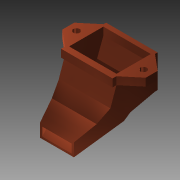
# Autodesk Inventor part: dysza_abs2
Saved by Autodesk Inventor 2013 (Build 170138000, 138)
## iProperties
Created: 2013-08-26
Part Number: dysza_abs2
Material: Generic
Document SubType Name: Modeling
Designer: dzban
Density: 1 g/cm^3
Author: dzban
Autodesk Inventor part; units mm, degrees
ref_plane "YZ Plane" through (0, 0, 0) normal (1, 0, 0) x (0, 1, 0)
ref_plane "XZ Plane" through (0, 0, 0) normal (0, 1, 0) x (-1, 0, 0)
ref_plane "XY Plane" through (0, 0, 0) normal (0, 0, 1) x (1, 0, 0)
sketch "Sketch1" plane through (0, 0, 0) normal (1, 0, 0) x (0, 1, 0)
  line L0 (0, 0) -> (15, 0)
  line L1 (15, 0) -> (12.3428, -7.0424)
  line L2 (12.3428, -7.0424) -> (2.9628, -13.5)
  line L3 (2.9628, -13.5) -> (-16.504, -16)
  line L4 (-16.504, -16) -> (-16.504, -11)
  line L5 (-16.504, -11) -> (-7.6685, -9.267)
  line L6 (-7.6685, -9.267) -> (-2.3251, -6.639)
  line L7 (-2.3251, -6.639) -> (0, 0)
  dimension "d0" = 15
  dimension "d24" = 16
  dimension "d27" = 5
  constraints: 16 end point, 1 horizontal, 1 vertical
  measures "d0" distance of L0.start L0.end
  measures "d24" distance from line of L0 L3.end
  measures "d27" distance of L3.end L4.end
extrude "Extrusion1" add sketch "Sketch1" along normal blind 20
sketch "Sketch2" plane through (0, 0, 0) normal (0, 0, 1) x (1, 0, 0)
  line L0 (-0.936, -0.2322) -> (7.6821, -18.3326)
  line L1 (7.6821, -18.3326) -> (-7.1135, -18.3326)
  line L2 (-7.1135, -18.3326) -> (-0.936, -0.2322)
  constraints: 6 end point
extrude "Extrusion2" cut sketch "Sketch2" against normal blind 25
shell "Shell1" thickness 0.8 removed faces 2 at (6.6667, 5, 0) at (11.2076, -16.504, -14.3333)
sketch "Sketch3" plane through (0, 0, 0) normal (0, 0, 1) x (1, 0, 0)
  line L0 (0.8, 0.8476) -> (0.8, 14.1449) projected
  line L1 (0.8, 14.1449) -> (19.2, 14.1449) projected
  line L2 (19.2, 14.1449) -> (19.2, 0.8476) projected
  line L3 (19.2, 0.8476) -> (0.8, 0.8476) projected
  line L4 (0, 0) -> (0, 15) projected
  line L5 (0, 0) -> (20, 0) projected
  line L6 (20, 15) -> (20, 0) projected
  line L7 (0, 15) -> (20, 15) projected
  circle A0 centre (-3, 7.5) radius 1.25
  circle A1 centre (23, 7.5) radius 1.25
  line L8 (0, 0) -> (-6.2, 5.2024)
  line L9 (-6.2, 5.2024) -> (-6.2, 9.7976)
  line L10 (-6.2, 9.7976) -> (0, 15)
  line L11 (20, 15) -> (26.2, 9.7976)
  line L12 (26.2, 9.7976) -> (26.2, 5.2024)
  line L13 (26.2, 5.2024) -> (20, 0)
  line L14 (0, 0) -> (0, -1.5)
  line L15 (0, -1.5) -> (20, -1.5)
  line L16 (20, -1.5) -> (20, 0)
  dimension "d6" = 2.5
  dimension "d8" = 2.5
  dimension "d9" = 3
  dimension "d10" = 3
  dimension "d11" = 7.5
  dimension "d12" = 7.5
  dimension "d17" = 130
  dimension "d18" = 130
  dimension "d19" = 130
  dimension "d20" = 130
  dimension "d21" = 6.2
  dimension "d22" = 6.2
  dimension "d23" = 1.5
  constraints: 18 end point, 2 centre point, 2 vertical, 1 horizontal
  measures "d6" diameter of A0
  measures "d8" diameter of A1
  measures "d9" distance from line of A0.centre L4
  measures "d10" distance from line of L6 A1.centre
  measures "d11" distance from line of L7 A0.centre
  measures "d12" distance from line of L7 A1.centre
  measures "d17" angle of L10 L9
  measures "d18" angle of L9 L8
  measures "d19" angle of L12 L11
  measures "d20" angle of L12 L13
  measures "d21" distance between parallel lines of L12 L6
  measures "d22" distance between parallel lines of L4 L9
  measures "d23" distance between parallel lines of L5 L15
extrude "Extrusion3" add sketch "Sketch3" along normal blind 3
sketch "Sketch4" plane through (20, 0, 0) normal (1, 0, 0) x (0, 0, -1)
  line L0 (13.5, 2.9628) -> (7.0424, 12.3428) projected
  line L1 (7.0424, 12.3428) -> (0, 15) projected
  line L2 (0, 15) -> (9.6524, 15)
  line L3 (9.6524, 15) -> (11.8288, 5.3904)
  constraints: 4 end point, 1 point on line
extrude "Extrusion4" add sketch "Sketch4" against normal blind 20
sketch "Sketch5" plane through (0, 15, 3) normal (0, 1, 0) x (1, 0, 0)
  line L0 (0, 3) -> (0, 0) projected
  line L1 (20, 0) -> (0, 0) projected
  line L2 (20, 3) -> (20, 0) projected
  line L3 (20, 12.6524) -> (20, 3) projected
  line L4 (20, 12.6524) -> (0, 12.6524) projected
  line L5 (0, 3) -> (0, 12.6524) projected
extrude "Extrusion5" add sketch "Sketch5" along normal blind 1
body "Solid1"
